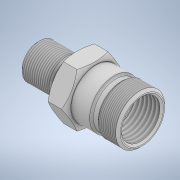
# Autodesk Inventor part: Штуцер
Saved by Autodesk Inventor 2021 (Build 250183000, 183)
## iProperties
Created: 2021-03-05
Part Number: Штуцер
Material: Типовые
Document SubType Name: Modeling
Designer: khosta
Density: 1 g/cm^3
Appearance: По умолчанию
Author: khosta
Autodesk Inventor part; units mm, degrees
ref_plane "YZ Plane" through (0, 0, 0) normal (1, 0, 0) x (0, 1, 0)
ref_plane "XZ Plane" through (0, 0, 0) normal (0, 1, 0) x (-1, 0, 0)
ref_plane "XY Plane" through (0, 0, 0) normal (0, 0, 1) x (1, 0, 0)
sketch "Эскиз1" plane through (0, 0, 0) normal (0, 0, 1) x (1, 0, 0)
  line L0 (0, 8) -> (0, 15.15)
  line L1 (32.7, 15.15) -> (32.7, 15.15)
  line L2 (31.1, 13.55) -> (27.1142, 13.55)
  line L3 (26.4071, 13.8429) -> (25.1, 15.15)
  line L4 (25.1, 15.15) -> (0, 15.15)
  line L5 (-18, 0) -> (108, 0) projected
  arc A0 (31.1, 13.55) -> (32.7, 15.15) centre (31.1, 15.15) ccw
  arc A1 (26.4071, 13.8429) -> (27.1142, 13.55) centre (27.1142, 14.55) ccw
  line L6 (0, 8) -> (59.8, 8)
  line L7 (65.7, 21) -> (50, 21)
  line L8 (50, 21) -> (50, 26.5)
  line L9 (65.7, 21) -> (65.7, 21)
  line L10 (67.3, 19.4) -> (71.2858, 19.4)
  line L11 (71.9929, 19.6929) -> (73.3, 21)
  line L12 (73.3, 21) -> (90, 21)
  arc A2 (65.7, 21) -> (67.3, 19.4) centre (67.3, 21) ccw
  arc A3 (71.2858, 19.4) -> (71.9929, 19.6929) centre (71.2858, 20.4) ccw
  line L13 (32.7, 15.15) -> (32.7, 26.5)
  line L14 (32.7, 26.5) -> (50, 26.5)
  line L15 (59.8, 8) -> (59.8, 16.5)
  line L16 (59.8, 16.5) -> (59.8, 16.5)
  line L17 (61.4, 18.1) -> (65.3858, 18.1)
  line L18 (66.0929, 17.8071) -> (67.4, 16.5)
  line L19 (67.4, 16.5) -> (90, 16.5)
  line L20 (90, 16.5) -> (90, 21)
  arc A4 (66.0929, 17.8071) -> (65.3858, 18.1) centre (65.3858, 17.1) ccw
  arc A5 (61.4, 18.1) -> (59.8, 16.5) centre (61.4, 16.5) ccw
  point P0 (0, 0)
  point P1 (32.7, 13.55)
  point P2 (26.7, 13.55)
  point P3 (65.7, 19.4)
  point P4 (71.7, 19.4)
  point P5 (59.8, 18.1)
  point P6 (65.8, 18.1)
  dimension "d0" = 8
  dimension "d1" = 7.15
  dimension "d2" = 32.7
  dimension "d4" = 1.6
  dimension "d5" = 6
  dimension "d6" = 135
  dimension "d7" = 13.55
  dimension "d9" = 1.6
  dimension "d10" = 1
  dimension "d11" = 59.8
  dimension "d14" = 24.3
  dimension "d15" = 1.6
  dimension "d16" = 6
  dimension "d17" = 135
  dimension "d18" = 19.4
  dimension "d19" = 1.6
  dimension "d20" = 1
  dimension "d22" = 30.2
  dimension "d24" = 26.5
  dimension "d25" = 1.6
  dimension "d26" = 6
  dimension "d27" = 135
  dimension "d28" = 1
  dimension "d29" = 1.6
  dimension "d30" = 90
  dimension "d31" = 21
  dimension "d32" = 16.5
  dimension "d33" = 18.1
  dimension "d34" = 8
  dimension "d35" = 40
  constraints: 40 end point, 12 point on circle, 12 point on line, 12 tangent, 6 centre point, 5 perpendicular, 4 horizontal, 4 vertical, 2 parallel
  measures "d0" distance of point (0, 0) L0.start
  measures "d1" distance of L0.start L0.end
  measures "d2" distance of L0.end L1.start
  measures "d4" distance of L1.start point (32.7, 13.55)
  measures "d5" distance of point (32.7, 13.55) point (26.7, 13.55)
  measures "d6" angle of L2 L3
  measures "d7" distance between parallel lines of L2 L5
  measures "d9" radius of A0
  measures "d10" radius of A1
  measures "d11" distance of L0.start L6.end
  measures "d14" distance of L12.end L7.start
  measures "d15" distance of L7.start point (65.7, 19.4)
  measures "d16" distance of point (65.7, 19.4) point (71.7, 19.4)
  measures "d17" angle of L11 L10
  measures "d18" distance between parallel lines of L5 L10
  measures "d19" radius of A2
  measures "d20" radius of A3
  measures "d22" distance of L19.end L15.end
  measures "d24" distance between parallel lines of L5 L14
  measures "d25" distance of L15.end point (59.8, 18.1)
  measures "d26" distance of point (59.8, 18.1) point (65.8, 18.1)
  measures "d27" angle of L17 L18
  measures "d28" radius of A4
  measures "d29" radius of A5
  measures "d30" angle of L15 L5
  measures "d31" distance between parallel lines of L12 L5
  measures "d32" distance between parallel lines of L19 L5
  measures "d33" distance between parallel lines of L17 L5
  measures "d34" distance between parallel lines of L6 L5
  measures "d35" distance between parallel lines of L8 L20
revolve "Вращение1" add sketch "Эскиз1" angle 360 about axis through (-10, 0, 0) along (1, 0, 0)
sketch "Эскиз2" plane through (0, 0, 0) normal (0, 1, 0) x (-1, 0, 0)
  line L0 (-32.7, 15.15) -> (-32.7, -15.15) projected
  line L1 (-32.7, 26.5) -> (-32.7, -26.5) projected
  line L2 (-32.7, 21.5) -> (-35.5868, 26.5)
  line L3 (-32.7, 21.5) -> (-26.9265, 21.5) construction
  line L4 (-32.7, 21.5) -> (-50, 21.5)
  line L5 (-50, 26.5) -> (-50, -26.5) projected
  line L6 (-50, 21.5) -> (-47.1132, 26.5)
  line L7 (-32.7, 26.5) -> (-50, 26.5) projected
  line L8 (-50, 21.5) -> (-44.2265, 21.5) construction
  line L9 (-47.1132, 26.5) -> (-50, 26.5)
  line L10 (-50, 26.5) -> (-50, 21.5)
  line L11 (-32.7, 21.5) -> (-32.7, 26.5)
  line L12 (-35.5868, 26.5) -> (-32.7, 26.5)
  line L13 (18, 0) -> (-108, 0) projected
  point P0 (0, 0)
  dimension "d38" = 120
  dimension "d39" = 60
  dimension "d45" = 21.5
  dimension "d46" = 26.5
  dimension "d47" = 2.8868
  constraints: 18 end point, 3 collinear, 3 horizontal, 3 point on line, 2 equal length
  measures "d38" angle of L3 L2
  measures "d39" angle of L8 L6
  measures "d45" distance between parallel lines of L13 L4
  measures "d46" distance from line of point (-35.587, 26.5) L13
  measures "d47" distance from line of point (-35.587, 26.5) L1
revolve "Вращение2" cut sketch "Эскиз2" angle 360 about axis through (-10, 0, 0) along (1, 0, 0) contours L2 L7 L1 | L5 L7 L6
sketch "Эскиз3" plane through (0, 0, 0) normal (1, 0, 0) x (0, 1, 0)
  line L0 (0, 26.5) -> (22.9497, 13.25)
  line L1 (22.9497, 13.25) -> (22.9497, -13.25)
  line L2 (22.9497, -13.25) -> (0, -26.5)
  line L3 (0, -26.5) -> (-22.9497, -13.25)
  line L4 (-22.9497, -13.25) -> (-22.9497, 13.25)
  line L5 (-22.9497, 13.25) -> (0, 26.5)
  line L6 (0, 34.2752) -> (29.6832, 17.1376)
  line L7 (29.6832, 17.1376) -> (29.6832, -17.1376)
  line L8 (29.6832, -17.1376) -> (0, -34.2752)
  line L9 (0, -34.2752) -> (-29.6832, -17.1376)
  line L10 (-29.6832, -17.1376) -> (-29.6832, 17.1376)
  line L11 (-29.6832, 17.1376) -> (0, 34.2752)
  point P0 (0, 0)
  point P1 (0, 0)
  point P2 (0, 0)
  point P3 (0, 0)
  dimension "d41" = 6.7335
  dimension "d42" = 52.6329
  constraints: 24 end point, 2 coincident, 1 parallel, 1 vertical, 26 other
  measures "d41" distance between parallel lines of L7 L1
  measures "d42" distance between parallel lines of L7 L4
extrude "Выдавливание1" cut sketch "Эскиз3" along normal blind 271
chamfer "Фаска1" distance 2 angle 45 1 edges at (90, -21, 0)
chamfer "Фаска2" distance 1.5 angle 45 1 edges at (90, -16.5, 0)
chamfer "Фаска3" distance 2 angle 45 1 edges at (0, -15.15, 0)
chamfer "Фаска4" distance 1 angle 45 1 edges at (0, -8, 0)
thread "Резьба1" size "G30.201x1.814" designation "G 7/8" class "A" standard "DIN Pipe Threads" length 27
thread "Резьба2" size "M42x1.5" class "6g" standard "ANSI Metric M Profile" length 27
thread "Резьба3" size "M33x3.5" class "6H" standard "ANSI Metric M Profile" length 27
